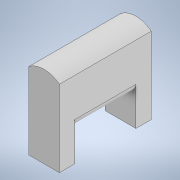
# Autodesk Inventor part: Odyssey Bushing
Saved by Autodesk Inventor 2021 (Build 250183000, 183)
## iProperties
Created: 2021-09-10
Part Number: Odyssey Bushing
Material: Generic
Document SubType Name: Modeling
Designer: Alex Clay
Density: 1 g/cm^3
Appearance: Default
Author: Alex Clay
Autodesk Inventor part; units mm, degrees
ref_plane "YZ Plane" through (0, 0, 0) normal (1, 0, 0) x (0, 1, 0)
ref_plane "XZ Plane" through (0, 0, 0) normal (0, 1, 0) x (-1, 0, 0)
ref_plane "XY Plane" through (0, 0, 0) normal (0, 0, 1) x (1, 0, 0)
sketch "Sketch1" plane through (0, 0, 0) normal (0, 0, 1) x (1, 0, 0)
  line L0 (-6.35, 31.75) -> (-6.35, 0)
  line L1 (-6.35, 0) -> (6.35, 0)
  line L2 (6.35, 0) -> (6.35, 31.75)
  arc A0 (6.35, 31.75) -> (-6.35, 31.75) centre (0, 23.8189) ccw
  point P0 (0, 0)
  dimension "d1" = 31.75
  dimension "d2" = 12.7
  dimension "d3" = 10.16
  constraints: 6 end point, 2 point on circle, 2 vertical, 1 centre point, 1 horizontal, 1 horizontal alignment, 1 midpoint, 1 vertical alignment
  measures "d1" distance of L1.end L2.end
  measures "d2" distance of L0.end L1.end
  measures "d3" radius of A0
extrude "Extrusion1" add sketch "Sketch1" along normal mid plane 38.1
sketch "Sketch2" plane through (0, 0, 0) normal (0, 0, 1) x (1, 0, 0)
  line L0 (-6.35, 0) -> (6.35, 0)
  line L1 (6.35, 0) -> (6.35, 12.7)
  line L2 (6.35, 12.7) -> (-6.35, 12.7)
  line L3 (-6.35, 12.7) -> (-6.35, 0)
  line L4 (0, -2.54) -> (0, 15.24) projected
  point P0 (0, 0)
  dimension "d6" = 12.7
  dimension "d7" = 6.35
  dimension "d10" = 12.7
  constraints: 8 end point, 2 parallel, 1 horizontal, 1 midpoint, 1 perpendicular
  measures "d6" distance of L0.start L0.end
  measures "d7" distance between parallel lines of L4 L1
  measures "d10" distance of L0.end L1.end
extrude "Extrusion2" cut sketch "Sketch2" along normal mid plane 25.4
fillet "Fillet1" radius 3.175 2 edges at (-6.35, 12.7, 0) (6.35, 12.7, 0)
equation "\"d7\" = 0.5 * d6"
body "Solid1"
